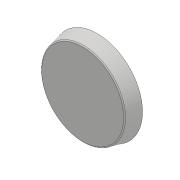
# Autodesk Inventor part: pot_holder_prototype
Saved by Autodesk Inventor 2017 (Build 210142000, 142)
## iProperties
Created: 2018-10-30
Part Number: pot_holder_prototype
Material: Generic
Document SubType Name: Modeling
Designer: mfans
Density: 1 g/cm^3
Appearance: Default
Author: mfans
Autodesk Inventor part; units mm, degrees
ref_plane "YZ Plane" through (0, 0, 0) normal (1, 0, 0) x (0, 1, 0)
ref_plane "XZ Plane" through (0, 0, 0) normal (0, 1, 0) x (-1, 0, 0)
ref_plane "XY Plane" through (0, 0, 0) normal (0, 0, 1) x (1, 0, 0)
sketch "Sketch1" plane through (0, 0, 0) normal (0, 0, 1) x (1, 0, 0)
  line L0 (0, 0) -> (37, 0)
  line L1 (37, 0) -> (40.0013, 13)
  line L2 (40.0013, 13) -> (0, 13)
  line L3 (0, 13) -> (0, 0)
  dimension "d0" = 77
  dimension "d2" = 37
  dimension "d3" = 13
  constraints: 8 end point, 1 horizontal, 1 parallel, 1 perpendicular
  measures "d0" angle of L0 L1
  measures "d2" distance of L0.start L0.end
  measures "d3" distance of L2.end L0.start
revolve "Revolution1" add sketch "Sketch1" angle 360 about axis through (0, 13, 0) along (0, -1, 0)
shell "Shell1" thickness 1.2 removed faces 1 at (-15.7395, 13, 6.8743)
fillet "Fillet1" radius 1 1 edges at (-36.0455, 1.2, 0)
fillet "Fillet2" radius 1 1 edges at (-37, 0, 0)
body "Solid1"
